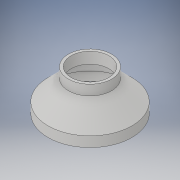
# Autodesk Inventor part: 4IN to 2IN D Adapter
Saved by Autodesk Inventor 2019 (Build 230136000, 136)
## iProperties
Created: 2019-01-05
Part Number: 4IN to 2IN D Adapter
Material: Generic
Document SubType Name: Modeling
Designer: alanl
Density: 1 g/cm^3
Appearance: Default
Author: alanl
Autodesk Inventor part; units mm, degrees
ref_plane "YZ Plane" through (0, 0, 0) normal (1, 0, 0) x (0, 1, 0)
ref_plane "XZ Plane" through (0, 0, 0) normal (0, 1, 0) x (-1, 0, 0)
ref_plane "XY Plane" through (0, 0, 0) normal (0, 0, 1) x (1, 0, 0)
sketch "Sketch1" plane through (0, 0, 0) normal (1, 0, 0) x (0, 1, 0)
  line L0 (50.8, 0) -> (-50.8, 0)
  line L1 (-13.5558, 52.4891) -> (-0.8558, 52.4891)
  line L2 (-0.8558, 52.4891) -> (24.5442, 27.0891)
  line L3 (24.5442, 27.0891) -> (37.2442, 27.0891)
  line L4 (37.2442, 23.7109) -> (23.1449, 23.7109)
  line L5 (23.1449, 23.7109) -> (-2.2551, 49.1109)
  line L6 (-2.2551, 49.1109) -> (-13.5558, 49.1109)
  line L7 (-13.5558, 52.4891) -> (-13.5558, 49.1109)
  line L8 (37.2442, 27.0891) -> (37.2442, 23.7109)
  point P0 (0, 0)
  dimension "d0" = 101.6
  dimension "d1" = 50.8
  dimension "d2" = 12.7
  dimension "d3" = 12.7
  dimension "d4" = 135
  dimension "d5" = 104.9782
  dimension "d6" = 54.1782
  dimension "d7" = 3.3782
  constraints: 18 end point, 3 parallel, 2 horizontal, 1 vertical, 2 other
  measures "d0" distance of L0.start L0.end
  measures "d1" distance of point (0, 0) L0.end
  measures "d2" distance of L1.start L1.end
  measures "d3" distance of L2.end L3.end
  measures "d4" angle of L1 L2
  measures "d5" diameter of L1 L0
  measures "d6" diameter of L3 L0
  measures "d7" distance between parallel lines of L2 L5
revolve "Revolution1" add sketch "Sketch1" angle 360 about axis through (0, 50.8, 0) along (0, -1, 0)
equation "\"d1\" = 0.5 * d0"
body "Solid1"
